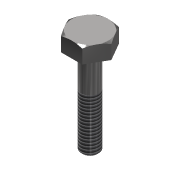
# Autodesk Inventor part: -
Saved by Autodesk Inventor 2021 (Build 250183000, 183)
## iProperties
Created: 2014-08-14
Part Number: -
Material: Stainless Steel
Document SubType Name: Modeling
Designer: dans
Mass: 268.56 g
Surface Area: 76.7287 cm^2
Volume: 33.2376 cm^3
Density: 8.08 g/cm^3
Appearance: Stainless - Polished
Description: HEAVY HEX STRUC BOLT-3/4"-10 UNC x 3.00"-ASTM A193-B8M (316)
Author: dans
Autodesk Inventor part; units mm, degrees
ref_plane "YZ Plane" through (0, 0, 0) normal (1, 0, 0) x (0, 1, 0)
ref_plane "XZ Plane" through (0, 0, 0) normal (0, 1, 0) x (-1, 0, 0)
ref_plane "XY Plane" through (0, 0, 0) normal (0, 0, 1) x (1, 0, 0)
sketch "Sketch1" plane through (0, 0, 0) normal (0, 1, 0) x (-1, 0, 0)
  line L0 (9.1654, 15.875) -> (18.3309, 0)
  line L1 (18.3309, 0) -> (9.1654, -15.875)
  line L2 (9.1654, -15.875) -> (-9.1654, -15.875)
  line L3 (-9.1654, -15.875) -> (-18.3309, 0)
  line L4 (-18.3309, 0) -> (-9.1654, 15.875)
  line L5 (-9.1654, 15.875) -> (9.1654, 15.875)
  point P0 (0, 0)
  point P1 (0, 0)
  dimension "HEX_FLATS" = 31.75
  constraints: 12 end point, 1 coincident, 1 horizontal, 13 other
  measures "HEX_FLATS" distance between parallel lines of L2 L5
extrude "Extrusion1" add sketch "Sketch1" along normal blind 13.3096
sketch "Sketch2" plane through (0, 0, 0) normal (0, 0, 1) x (1, 0, 0)
  line L0 (9.1654, 13.3096) -> (18.3309, 13.3096) projected
  line L1 (15.875, 13.3096) -> (28.575, 5.9773)
  line L2 (28.575, 5.9773) -> (28.575, 18.6773)
  line L3 (28.575, 18.6773) -> (15.875, 18.6773)
  line L4 (15.875, 18.6773) -> (15.875, 13.3096)
  line L5 (0, 26.9922) -> (0, -31.2125) projected
  line L6 (0, 0) -> (0, -22.8975)
  dimension "d3" = 30
  dimension "HD_CHAMFER" = 15.875
  dimension "d5" = 12.7
  dimension "d6" = 12.7
  constraints: 10 end point, 2 point on line, 2 vertical, 1 horizontal
  measures "d3" angle of L1 L0
  measures "HD_CHAMFER" distance between parallel lines of L4 L5
  measures "d5" distance of L2.end L3.end
  measures "d6" distance of L1.end L2.end
revolve "Revolution1" cut sketch "Sketch2" angle 360 about axis through (0, 0, 0) along (0, -1, 0)
sketch "Sketch3" plane through (0, 0, 0) normal (0, -1, 0) x (1, 0, 0)
  circle A0 centre (0, 0) radius 7.5
  dimension "BOLT_SIZE" = 15
  constraints: 1 centre point, 1 coincident
  measures "BOLT_SIZE" diameter of A0
extrude "Extrusion2" add sketch "Sketch3" along normal blind 76.2
chamfer "Chamfer1" distance 1.524 angle 45 1 edges at (-7.5, -76.2, 0)
thread "Thread 1/2\"" size "1/2-13 UNC" class "2A" standard "ANSI Unified Screw Threads" length 0
thread "Thread 5/8\"" size "5/8-11 UNC" class "2A" standard "ANSI Unified Screw Threads" length 0
thread "Thread-3/4\"" size "3/4-10 UNC" class "2A" standard "ANSI Unified Screw Threads" length 44.45
thread "Thread 7/8\"" size "7/8-9 UNC" class "2A" standard "ANSI Unified Screw Threads" length 0
thread "Thread 1\"" size "1-8 UNC" class "2A" standard "ANSI Unified Screw Threads" length 0
thread "Thread 1 1/8\"" size "1 1/8-7 UNC" class "2A" standard "ANSI Unified Screw Threads" length 0
thread "Thread 1 1/4\"" size "1 1/4-7 UNC" class "2A" standard "ANSI Unified Screw Threads" length 0
body "Solid1"
